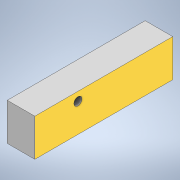
# Autodesk Inventor part: SLIDERCRANK-BASE CUBOID
Saved by Autodesk Inventor 2021 (Build 250183000, 183)
## iProperties
Created: 2021-07-25
Part Number: SLIDERCRANK-BASE CUBOID
Material: Generic
Document SubType Name: Modeling
Designer: HP
Density: 1 g/cm^3
Appearance: Default
Author: HP
Autodesk Inventor part; units mm, degrees
ref_plane "YZ Plane" through (0, 0, 0) normal (1, 0, 0) x (0, 1, 0)
ref_plane "XZ Plane" through (0, 0, 0) normal (0, 1, 0) x (-1, 0, 0)
ref_plane "XY Plane" through (0, 0, 0) normal (0, 0, 1) x (1, 0, 0)
sketch "Sketch1" plane through (0, 0, 0) normal (1, 0, 0) x (0, 1, 0)
  point P0 (0, 0)
sketch "Sketch2" plane through (0, 0, 0) normal (1, 0, 0) x (0, 1, 0)
  line L0 (9.525, 39.6875) -> (-11.1252, 39.6875)
  line L1 (-11.1252, 39.6875) -> (-11.1252, -36.5125)
  line L2 (-11.1252, -36.5125) -> (9.525, -36.5125)
  line L3 (9.525, -36.5125) -> (9.525, 39.6875)
  line L4 (9.525, -22.225) -> (9.525, -36.5125)
  point P0 (0, 0)
  dimension "d0" = 20.6502
  dimension "d1" = 76.2
  constraints: 10 end point, 2 parallel, 1 horizontal, 1 perpendicular
  measures "d0" distance of L2.end L1.end
  measures "d1" distance of L1.end L0.end
extrude "Extrusion1" add sketch "Sketch2" along normal blind 15.24
sketch "Sketch3" plane through (15.24, 0, 0) normal (1, 0, 0) x (0, 0, -1)
  circle A0 centre (-15.875, 4.7625) radius 2.2479
  point P0 (0, 0)
  dimension "d4" = 4.4958
  constraints: 1 centre point
  measures "d4" diameter of A0
extrude "Extrusion2" cut sketch "Sketch3" along normal mid plane 50.8
body "Solid1"
